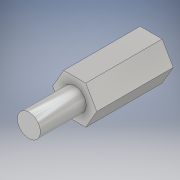
# Autodesk Inventor part: Spacer7mm_m3
Saved by Autodesk Inventor 2019 (Build 230136000, 136)
## iProperties
Created: 2020-02-24
Part Number: Spacer7mm_m3
Material: Generic
Document SubType Name: Modeling
Designer: lgnds
Density: 1 g/cm^3
Appearance: Default
Author: lgnds
Autodesk Inventor part; units mm, degrees
ref_plane "YZ Plane" through (0, 0, 0) normal (1, 0, 0) x (0, 1, 0)
ref_plane "XZ Plane" through (0, 0, 0) normal (0, 1, 0) x (-1, 0, 0)
ref_plane "XY Plane" through (0, 0, 0) normal (0, 0, 1) x (1, 0, 0)
sketch "Sketch1" plane through (0, 0, 0) normal (0, 0, 1) x (1, 0, 0)
  line L0 (2.8868, 0) -> (1.4434, -2.5)
  line L1 (1.4434, -2.5) -> (-1.4434, -2.5)
  line L2 (-1.4434, -2.5) -> (-2.8868, 0)
  line L3 (-2.8868, 0) -> (-1.4434, 2.5)
  line L4 (-1.4434, 2.5) -> (1.4434, 2.5)
  line L5 (1.4434, 2.5) -> (2.8868, 0)
  point P0 (0, 0)
  point P1 (0, 0)
  dimension "d0" = 5
  constraints: 12 end point, 1 coincident, 1 horizontal, 13 other
  measures "d0" distance between parallel lines of L4 L1
extrude "Extrusion1" add sketch "Sketch1" along normal blind 10
sketch "Sketch2" plane through (0, 0, 10) normal (0, 0, 1) x (1, 0, 0)
  circle A0 centre (0, 0) radius 1.5
  dimension "d3" = 3
  constraints: 1 centre point, 1 coincident
  measures "d3" diameter of A0
extrude "Extrusion2" add sketch "Sketch2" along normal blind 6
sketch "Sketch3" plane through (0, 0, 0) normal (0, 0, -1) x (-1, 0, 0)
  circle A0 centre (0, 0) radius 1.5
  dimension "d6" = 3
  constraints: 1 centre point, 1 coincident
  measures "d6" diameter of A0
extrude "Extrusion3" cut sketch "Sketch3" against normal blind 4
body "Solid1"
